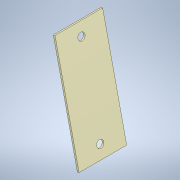
# Autodesk Inventor part: アームガード
Saved by Autodesk Inventor 2020.2 (Build 242310000, 310)
## iProperties
Created: 2020-03-29
Part Number: アームガード
Material: ポリプロピレン
Document SubType Name: Modeling
Designer: aoyama
Density: 0.899 g/cm^3
Appearance: 滑らか - 灰色
Author: aoyama
Autodesk Inventor part; units mm, degrees
ref_plane "YZ Plane" through (0, 0, 0) normal (1, 0, 0) x (0, 1, 0)
ref_plane "XZ Plane" through (0, 0, 0) normal (0, 1, 0) x (-1, 0, 0)
ref_plane "XY Plane" through (0, 0, 0) normal (0, 0, 1) x (1, 0, 0)
sketch "スケッチ1" plane through (0, 0, 0) normal (0, 0, 1) x (1, 0, 0)
  circle A0 centre (54.6996, 44) radius 4
  line L0 (61.9927, 0) -> (64.9927, 0)
  line L1 (58.602, 44.878) -> (68.6996, 0)
  line L2 (64.9927, 0) -> (67.602, 4.878)
  line L3 (59.3337, 45.0427) -> (69.4313, 0.1646)
  line L4 (59.3337, 45.0427) -> (58.602, 44.878)
  line L5 (68.6996, 0) -> (69.4313, 0.1646)
  point P0 (0, 0)
  dimension "d0" = 5
  dimension "d1" = 0.75
  dimension "d12" = 77.32
  constraints: 12 end point, 2 perpendicular, 1 horizontal, 1 parallel, 1 point on line, 8 other
  measures "d0" distance of L1.end L2.end
  measures "d1" distance between parallel lines of L1 L3
  measures "d12" angle of L1 L0
extrude "押し出し1" add sketch "スケッチ1" along normal blind 20 contours L4 L3 L5 L1
sketch "スケッチ2" plane through (59.3337, 45.0427, 20) normal (0.9756, 0.2195, 0) x (0, 0, -1)
  line L0 (20, -46) -> (20, 0) projected
  line L1 (20, 0) -> (0, 0) projected
  line L2 (0, -46) -> (0, 0) projected
  line L3 (20, -46) -> (0, -46) projected
  circle A0 centre (10, -41) radius 1.5
  circle A1 centre (10, -5) radius 1.5
  point P0 (20, -30.9196)
  dimension "d4" = 3
  dimension "d5" = 5
  dimension "d6" = 10
  dimension "d7" = 3
  dimension "d8" = 5
  dimension "d9" = 10
  constraints: 2 centre point
  measures "d4" diameter of A0
  measures "d5" distance from line of L3 A0.centre
  measures "d6" distance from line of L0 A0.centre
  measures "d7" diameter of A1
  measures "d8" distance from line of L1 A1.centre
  measures "d9" distance from line of L0 A1.centre
extrude "押し出し2" cut sketch "スケッチ2" against normal blind 0.75 contours A0 | A1
